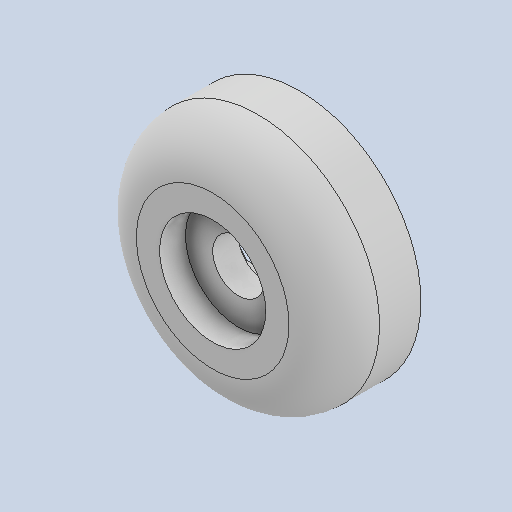
# Autodesk Inventor part: TTencodercap
Saved by Autodesk Inventor 2022 (Build 260153070, 153G)
## iProperties
Created: 2021-11-27
Part Number: TTencodercap
Material: Generic
Document SubType Name: Modeling
Designer: a laptop
Density: 1 g/cm^3
Appearance: Default
Author: a laptop
Autodesk Inventor part; units mm, degrees
ref_plane "YZ Plane" through (0, 0, 0) normal (1, 0, 0) x (0, 1, 0)
ref_plane "XZ Plane" through (0, 0, 0) normal (0, 1, 0) x (-1, 0, 0)
ref_plane "XY Plane" through (0, 0, 0) normal (0, 0, 1) x (1, 0, 0)
sketch "Sketch1" plane through (0, 0, 0) normal (0, 0, 1) x (1, 0, 0)
  circle A0 centre (0, 0) radius 4.7 projected
  circle A1 centre (0, 0) radius 1 projected
  line L0 (-2.0304, 2) -> (2.0304, 2) projected
  arc A2 (-2.0304, 2) -> (-2.0304, -2) centre (0, 0) ccw projected
  arc A3 (2.0304, -2) -> (2.0304, 2) centre (0, 0) ccw projected
  line L1 (2.0304, -2) -> (-2.0304, -2) projected
ref_plane "Work Plane1" through (-12.875, -12.875, -1.15) normal (0, 0, 1) x (1, 0, 0)
extrude "Extrusion1" add sketch "Sketch1" along normal blind 0.2 and the other way blind 1.15 contours A0
sketch "Sketch2" plane through (0, 0, 0.2) normal (0, 0, 1) x (1, 0, 0)
  circle A0 centre (0, 0) radius 4.7 projected
  circle A1 centre (0, 0) radius 1 projected
extrude "Extrusion2" add sketch "Sketch2" along normal blind 2
fillet "Fillet1" radius 1.75 1 edges at (-4.7, 0, 2.2)
sketch "Sketch3" plane through (0, 0, 2.2) normal (0, 0, 1) x (1, 0, 0)
  circle A0 centre (0, 0) radius 2.05
  circle A1 centre (0, 0) radius 1 projected
  point P0 (0, 0)
  dimension "d7" = 4.1
  constraints: 1 centre point, 1 concentric
  measures "d7" diameter of A0
extrude "Extrusion3" cut sketch "Sketch3" against normal blind 1 contours A0 | A1
body "Solid1"
